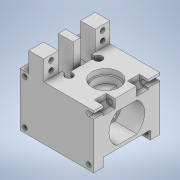
# Autodesk Inventor part: YCarriage
Saved by Autodesk Inventor 2020 (Build 240168000, 168)
## iProperties
Created: 2022-04-26
Part Number: YCarriage
Material: Ogólny
Document SubType Name: Modeling
Designer: mikoma
Density: 1 g/cm^3
Appearance: Domyślna
Author: mikoma
Autodesk Inventor part; units mm, degrees
ref_plane "YZ Plane" through (0, 0, 0) normal (1, 0, 0) x (0, 1, 0)
ref_plane "XZ Plane" through (0, 0, 0) normal (0, 1, 0) x (-1, 0, 0)
ref_plane "XY Plane" through (0, 0, 0) normal (0, 0, 1) x (1, 0, 0)
sketch "Szkic1" plane through (0, 0, 0) normal (0, 1, 0) x (-1, 0, 0)
  line L0 (-50, 45) -> (50, 45)
  line L1 (50, 45) -> (50, -45)
  line L2 (50, -45) -> (-50, -45)
  line L3 (-50, -45) -> (-50, 45)
  line L4 (-50, 45) -> (50, -45) construction
  line L5 (50, 45) -> (-50, -45) construction
  point P0 (0, 0)
  dimension "d0" = 90
  dimension "d1" = 100
  constraints: 12 end point, 2 midpoint, 2 parallel, 1 horizontal, 1 perpendicular
  measures "d0" distance of L0.end L1.end
  measures "d1" distance between parallel lines of L1 L3
extrude "Wyciągnięcie proste1" add sketch "Szkic1" along normal blind 73
sketch "Szkic2" plane through (-50, 0, 45) normal (0, 0, 1) x (1, 0, 0)
  circle A0 centre (6.5, 66.5) radius 3.25
  circle A1 centre (93.5, 66.5) radius 3.25
  circle A2 centre (6.5, 6.5) radius 3.25
  circle A3 centre (93.5, 6.5) radius 3.25
  line L0 (0, 0) -> (0, 73) projected
  line L1 (0, 73) -> (100, 73) projected
  line L2 (0, 0) -> (100, 0) projected
  line L3 (100, 0) -> (100, 73) projected
  circle A4 centre (6.5, 66.5) radius 5.5
  circle A5 centre (6.5, 6.5) radius 5.5
  circle A6 centre (93.5, 6.5) radius 5.5
  circle A7 centre (93.5, 66.5) radius 5.5
  line L4 (12, 66.5) -> (12, 73)
  line L5 (6.5, 61) -> (0, 61)
  line L6 (0, 0) -> (0, 73) projected
  line L7 (6.5, 12) -> (0, 12)
  line L8 (12, 6.5) -> (12, 0)
  line L9 (100, 0) -> (0, 0) projected
  line L10 (93.5, 12) -> (100, 12)
  line L11 (88, 6.5) -> (88, 0)
  line L12 (88, 66.5) -> (88, 73)
  line L13 (100, 73) -> (0, 73) projected
  line L14 (93.5, 61) -> (100, 61)
  line L15 (0, 73) -> (12, 73)
  line L16 (12, 73) -> (12, 61)
  line L17 (12, 61) -> (0, 61)
  line L18 (0, 61) -> (0, 73)
  point P0 (50, 0)
  point P1 (12, 0)
  point P2 (6.5, 61)
  point P3 (12, 66.5)
  dimension "d4" = 6.5
  dimension "d5" = 6.5
  dimension "d6" = 6.5
  dimension "d7" = 6.5
  dimension "d8" = 6.5
  dimension "d9" = 6.5
  dimension "d10" = 11
  constraints: 24 end point, 9 perpendicular, 8 centre point, 8 point on circle, 8 point on line, 8 tangent, 6 equal radius, 4 coincident, 3 horizontal alignment, 2 parallel, 2 vertical alignment, 1 horizontal
  measures "d4" distance from line of L0 A0.centre
  measures "d5" distance from line of L1 A0.centre
  measures "d6" distance from line of L0 A2.centre
  measures "d7" distance from line of L2 A2.centre
  measures "d8" diameter of A0
  measures "d9" distance from line of L3 A1.centre
  measures "d10" diameter of A4
ref_plane "Płaszczyzna konstrukcyjna1" through (-50, 0, 32) normal (0, 0, 1) x (1, 0, 0)
extrude "Wyciągnięcie proste2" cut sketch "Szkic2" against normal blind 64 from surface at -13 contours A0 | A2 | A3 | L0 L7 A5 L8 L2 | L0 L1 L4 A4 L5 | A5 | L11 A6 L10 L3 L2 | A4 | A4 L16 L17 | A6
extrude "Wyciągnięcie proste3" cut sketch "Szkic2" against normal through all contours A0 | A1 | A2 | A3
sketch "Szkic3" plane through (50, 0, 45) normal (1, 0, 0) x (0, 0, -1)
  circle A0 centre (45, 36.5) radius 14.25
  line L0 (77, 0) -> (90, 0) projected
  circle A1 centre (45, 36.5) radius 24.25
  line L1 (31.2864, 56.5) -> (58.7136, 56.5)
  line L2 (31.2864, 16.5) -> (58.7136, 16.5)
  circle A2 centre (45, 36.5) radius 19 construction
  circle A3 centre (26, 36.5) radius 2.75
  circle A4 centre (31.565, 49.935) radius 2.75
  circle A5 centre (31.565, 23.065) radius 2.75
  circle A6 centre (58.435, 23.065) radius 2.75
  circle A7 centre (64, 36.5) radius 2.75
  circle A8 centre (58.435, 49.935) radius 2.75
  line L3 (31.565, 23.065) -> (45, 36.5) construction
  line L4 (31.565, 49.935) -> (45, 36.5) construction
  line L5 (45, 36.5) -> (26, 36.5) construction
  line L6 (29.2556, 53.935) -> (33.8744, 53.935)
  line L7 (33.8744, 53.935) -> (36.1838, 49.935)
  line L8 (36.1838, 49.935) -> (33.8744, 45.935)
  line L9 (33.8744, 45.935) -> (29.2556, 45.935)
  line L10 (29.2556, 45.935) -> (26.9462, 49.935)
  line L11 (26.9462, 49.935) -> (29.2556, 53.935)
  line L12 (30, 38.8094) -> (30, 34.1906)
  line L13 (30, 34.1906) -> (26, 31.8812)
  line L14 (26, 31.8812) -> (22, 34.1906)
  line L15 (22, 34.1906) -> (22, 38.8094)
  line L16 (22, 38.8094) -> (26, 41.1188)
  line L17 (26, 41.1188) -> (30, 38.8094)
  line L18 (29.2556, 27.065) -> (33.8744, 27.065)
  line L19 (33.8744, 27.065) -> (36.1838, 23.065)
  line L20 (36.1838, 23.065) -> (33.8744, 19.065)
  line L21 (33.8744, 19.065) -> (29.2556, 19.065)
  line L22 (29.2556, 19.065) -> (26.9462, 23.065)
  line L23 (26.9462, 23.065) -> (29.2556, 27.065)
  line L24 (63.0538, 23.065) -> (60.7444, 19.065)
  line L25 (60.7444, 19.065) -> (56.1256, 19.065)
  line L26 (56.1256, 19.065) -> (53.8162, 23.065)
  line L27 (53.8162, 23.065) -> (56.1256, 27.065)
  line L28 (56.1256, 27.065) -> (60.7444, 27.065)
  line L29 (60.7444, 27.065) -> (63.0538, 23.065)
  line L30 (64, 41.1188) -> (68, 38.8094)
  line L31 (68, 38.8094) -> (68, 34.1906)
  line L32 (68, 34.1906) -> (64, 31.8812)
  line L33 (64, 31.8812) -> (60, 34.1906)
  line L34 (60, 34.1906) -> (60, 38.8094)
  line L35 (60, 38.8094) -> (64, 41.1188)
  line L36 (56.1256, 53.935) -> (60.7444, 53.935)
  line L37 (60.7444, 53.935) -> (63.0538, 49.935)
  line L38 (63.0538, 49.935) -> (60.7444, 45.935)
  line L39 (60.7444, 45.935) -> (56.1256, 45.935)
  line L40 (56.1256, 45.935) -> (53.8162, 49.935)
  line L41 (53.8162, 49.935) -> (56.1256, 53.935)
  circle A9 centre (45, 36.5) radius 10
  point P0 (45, 0)
  dimension "d16" = 36.5
  dimension "d17" = 45
  dimension "d18" = 28.5
  dimension "d19" = 48.5
  dimension "d20" = 40
  dimension "d21" = 20
  dimension "d22" = 38
  dimension "d23" = 5.5
  dimension "d24" = 45
  dimension "d25" = 45
  dimension "d26" = 8
  dimension "d27" = 8
  dimension "d28" = 8
  dimension "d29" = 8
  dimension "d30" = 8
  dimension "d31" = 8
  dimension "d32" = 20
  constraints: 82 end point, 10 centre point, 10 coincident, 10 point on circle, 6 horizontal, 5 equal radius, 3 point on line, 2 vertical, 1 parallel, 78 other
  measures "d16" distance from line of L0 A0.centre
  measures "d17" horizontal distance of L0.end A0.centre
  measures "d18" diameter of A0
  measures "d19" diameter of A1
  measures "d20" distance between parallel lines of L2 L1
  measures "d21" distance from line of L1 A0.centre
  measures "d22" diameter of A2
  measures "d23" diameter of A4
  measures "d24" angle of L4 L5
  measures "d25" angle of L5 L3
  measures "d26" distance between parallel lines of L9 L6
  measures "d27" distance between parallel lines of L12 L15
  measures "d28" distance between parallel lines of L21 L18
  measures "d29" distance between parallel lines of L25 L28
  measures "d30" distance between parallel lines of L36 L39
  measures "d31" distance between parallel lines of L31 L34
  measures "d32" diameter of A9
extrude "Wyciągnięcie proste4" cut sketch "Szkic3" against normal blind 30 contours A0 | A1 L2 L1 | A3 | A4 | A5 | A6 | A7 | A8 | L6 L7 L8 L9 L10 L11 | L12 L13 L14 L15 L16 L17 | L18 L19 L20 L21 L22 L23 | L24 L25 L26 L27 L28 L29 | L30 L31 L32 L33 L34 L35 | L36 L37 L38 L39 L40 L41 | A9
extrude "Wyciągnięcie proste5" cut sketch "Szkic3" against normal blind 85 contours A0 | A9
extrude "Wyciągnięcie proste6" cut sketch "Szkic3" against normal through all contours A3 | A4 | A5 | A6 | A7 | A8 | A9
extrude "Wyciągnięcie proste7" cut sketch "Szkic3" along normal blind 20 from surface at -100 contours A3 | A4 | A5 | A6 | A7 | A8 | L6 L7 L8 L9 L10 L11 | L12 L13 L14 L15 L16 L17 | L18 L19 L20 L21 L22 L23 | L24 L25 L26 L27 L28 L29 | L30 L31 L32 L33 L34 L35 | L36 L37 L38 L39 L40 L41
sketch "Szkic4" plane through (0, 73, 0) normal (0, 1, 0) x (1, 0, 0)
  line L0 (-18, -5) -> (-18, -25)
  line L1 (-18, -25) -> (-38, -25)
  line L2 (-38, -25) -> (-38, -5)
  line L3 (-38, -5) -> (-18, -5)
  line L4 (-18, 25) -> (-18, 5)
  line L5 (-18, 5) -> (-38, 5)
  line L6 (-38, 5) -> (-38, 25)
  line L7 (-38, 25) -> (-18, 25)
  line L8 (-38, 32) -> (-38, -32) projected
  arc A0 (-12, 16.0869) -> (-10.7084, 15.2371) centre (-8.5, 20) ccw construction
  arc A1 (-13.744, -20.25) -> (-10.7084, -15.2371) centre (-8.5, -20) ccw
  line L9 (-18, 20.25) -> (-18, -20.25)
  line L10 (-18, -20.25) -> (-13.744, -20.25)
  line L11 (-12, -20.25) -> (-12, -16.0869) construction
  line L12 (-12, 20.25) -> (-13.744, 20.25) construction
  line L13 (-12, 16.0869) -> (-12, 20.25) construction
  line L14 (-13.744, 20.25) -> (-18, 20.25)
  line L15 (-13.744, -20.25) -> (-12, -20.25) construction
  line L16 (-12, -16.0869) -> (-12, -13) construction
  arc A2 (-13.744, 20.25) -> (-12, 16.0869) centre (-8.5, 20) ccw construction
  arc A3 (-12, -16.0869) -> (-13.744, -20.25) centre (-8.5, -20) ccw construction
  line L17 (-10.7084, -15.2371) -> (-12, -13)
  line L18 (-12, 13) -> (-10.7084, 15.2371)
  arc A4 (-10.7084, 15.2371) -> (-13.744, 20.25) centre (-8.5, 20) ccw
  line L19 (-12, 13) -> (-12, 16.0869) construction
  arc A5 (-10.7084, -15.2371) -> (-12, -16.0869) centre (-8.5, -20) ccw construction
  line L20 (-12, -13) -> (-12, 13)
  circle A6 centre (21.5, 0) radius 18.5
  circle A7 centre (21.5, 0) radius 16.5
  line L21 (50, 45) -> (-50, 45) projected
  line L22 (-50, -45) -> (50, -45) projected
  line L23 (-38, 45) -> (-18, 45)
  line L24 (-18, 45) -> (-18, -45)
  line L25 (-18, -45) -> (-38, -45)
  line L26 (-38, -45) -> (-38, 45)
  line L27 (20, -13.7136) -> (20, 13.7136) projected
  line L28 (20, 18.4391) -> (20, -18.4391)
  point P0 (0, 0)
  point P1 (-28, -15)
  point P2 (-28, 15)
  point P3 (-69.5, 24.5)
  point P4 (-18, 5)
  point P5 (20, 16.4317)
  point P6 (20, -16.4317)
  dimension "d41" = 20
  dimension "d42" = 20
  dimension "d43" = 5
  dimension "d44" = 5
  dimension "d45" = 10.5
  dimension "d46" = 6
  dimension "d47" = 3.5
  dimension "d48" = 150
  dimension "d49" = 150
  dimension "d50" = 26
  dimension "d51" = 40
  dimension "d53" = 5.244
  dimension "d54" = 7
  dimension "d55" = 0.25
  dimension "d56" = 0.25
  dimension "d57" = 20
  dimension "d58" = 59.5
  dimension "d59" = 37
  dimension "d60" = 33
  constraints: 50 end point, 14 point on circle, 9 parallel, 8 centre point, 5 point on line, 5 vertical alignment, 3 perpendicular, 2 vertical, 1 coincident, 1 equal radius, 1 horizontal, 1 horizontal alignment, 18 other
  measures "d41" distance of L1.end L2.end
  measures "d42" distance of L5.end L6.end
  measures "d43" vertical distance of point (0, 0) L5.end
  measures "d44" distance from line of point (0, 0) L3
  measures "d45" diameter of A0
  measures "d46" distance of L13.end L9.start
  measures "d47" distance from line of L11 A0.centre
  measures "d48" angle of L17 L16
  measures "d49" angle of L16 L18
  measures "d50" distance of L20.start L20.end
  measures "d51" distance of A5.centre A0.centre
  measures "d53" horizontal distance of L15.start A5.centre
  measures "d54" vertical distance of A5.centre L20.start
  measures "d55" distance from line of L10 A5.centre
  measures "d56" distance from line of L14 A0.centre
  measures "d57" vertical distance of point (0, 0) A5.centre
  measures "d58" distance from line of L2 A6.centre
  measures "d59" diameter of A6
  measures "d60" diameter of A7
extrude "Wyciągnięcie proste8" cut sketch "Szkic4" against normal blind 18 contours L9 L4 L14 A4 L18 L20 L17 A1 L10 L0 | L0 L1 L2 L3 | L5 L6 L7 L4
extrude "Wyciągnięcie proste9" cut sketch "Szkic4" against normal up to surface (16.5 mm away) contours L28 L27 A7 | A7 L28 L27
extrude "Wyciągnięcie proste10" cut sketch "Szkic4" against normal blind 22 contours A7 L28 L27 picked at (26, 0)
extrude "Wyciągnięcie proste11" cut sketch "Szkic4" against normal blind 7 contours A6 L28 A7 | L28 A7 A6
extrude "Wyciągnięcie proste12" cut sketch "Szkic2" against normal blind 16 from surface at -13 contours L1 L3 L14 A7 L12 | A7
ref_plane "Płaszczyzna konstrukcyjna2" through (50, 73, -29) normal (0, 0, -1) x (-1, 0, 0)
extrude "Wyciągnięcie proste13" cut sketch "Szkic2" along normal blind 16 from surface at -74 contours A1 | L1 L3 L14 A7 L12 | A7
sketch "Szkic5" plane through (50, 0, 45) normal (1, 0, 0) x (0, 0, -1)
  line L0 (13, 63.25) -> (13, 69.75) projected
  line L1 (58, 69.75) -> (58, 63.25) projected
  line L2 (0, 63.25) -> (0, 69.75) projected
  line L3 (13, 69.75) -> (0, 69.75)
  line L4 (0, 69.75) -> (0, 63.25)
  line L5 (0, 63.25) -> (13, 63.25)
  line L6 (13, 63.25) -> (13, 69.75)
  line L7 (74, 69.75) -> (74, 63.25) projected
  line L8 (90, 0) -> (90, 73) projected
  line L9 (74, 69.75) -> (90, 69.75)
  line L10 (90, 69.75) -> (90, 63.25)
  line L11 (90, 63.25) -> (74, 63.25)
  line L12 (74, 63.25) -> (74, 69.75)
  point P0 (45, 0)
  constraints: 16 end point, 4 parallel, 2 horizontal, 2 perpendicular, 1 horizontal alignment, 1 point on line
extrude "Wyciągnięcie proste14" cut sketch "Szkic5" against normal up to surface round surface about axis through (43.5, 66.5, 45) along (0, 0, -1) radius 3.25 far side no
extrude "Wyciągnięcie proste15" add sketch "Szkic4" along normal blind 27 contours L3 L8 L5 L9 | L24 L22 L26 L8 L1 | L8 L26 L21 L24 L7
sketch "Szkic6" plane through (-38, 61, -32) normal (-1, 0, 0) x (0, 0, 1)
  circle A0 centre (-3, 32.5) radius 3.25
  circle A1 centre (-3, 20.5) radius 3.25
  line L0 (-13, 39) -> (7, 39) projected
  line L1 (-13, 12) -> (-13, 39) projected
  circle A2 centre (67, 32.5) radius 3.25
  circle A3 centre (67, 20.5) radius 3.25
  line L2 (77, 12) -> (77, 39) projected
  line L3 (57, 39) -> (77, 39) projected
  point P0 (32, -61)
  dimension "d78" = 6.5
  dimension "d79" = 6.5
  dimension "d80" = 10
  dimension "d81" = 12
  dimension "d82" = 10
  dimension "d83" = 6.5
  dimension "d84" = 12
  constraints: 4 centre point, 3 equal radius, 2 vertical alignment
  measures "d78" diameter of A0
  measures "d79" distance from line of L0 A0.centre
  measures "d80" distance from line of L1 A0.centre
  measures "d81" distance of A0.centre A1.centre
  measures "d82" distance from line of L2 A2.centre
  measures "d83" distance from line of L3 A2.centre
  measures "d84" distance of A2.centre A3.centre
extrude "Wyciągnięcie proste16" cut sketch "Szkic6" against normal through all
equation "\"d21\" = 0.5 * d20"
equation "\"d27\" = d26"
equation "\"d28\" = d26"
equation "\"d29\" = d26"
equation "\"d30\" = d26"
equation "\"d31\" = d26"
